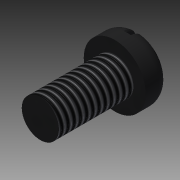
# Autodesk Inventor part: M3 6mm screw
Saved by Autodesk Inventor 2015 (Build 190159000, 159)
## iProperties
Created: 2015-10-31
Part Number: M3 6mm screw
Material: Nylon 6
Document SubType Name: Modeling
Designer: James
Density: 1.12 g/cm^3
Appearance: Nylon 6
Author: James
Autodesk Inventor part; units mm, degrees
ref_plane "YZ Plane" through (0, 0, 0) normal (1, 0, 0) x (0, 1, 0)
ref_plane "XZ Plane" through (0, 0, 0) normal (0, 1, 0) x (-1, 0, 0)
ref_plane "XY Plane" through (0, 0, 0) normal (0, 0, 1) x (1, 0, 0)
sketch "Sketch1" plane through (0, 0, 0) normal (0, 1, 0) x (-1, 0, 0)
  circle A0 centre (0, 0) radius 2.5
  dimension "d0" = 5
  constraints: 1 centre point, 1 coincident
  measures "d0" diameter of A0
extrude "Extrusion1" add sketch "Sketch1" along normal blind 2
fillet "Fillet1" radius 1 1 edges at (2.5, 2, 0)
sketch "Sketch2" plane through (0, 0, 0) normal (0, -1, 0) x (1, 0, 0)
  circle A0 centre (0, 0) radius 1.5
  constraints: 1 centre point, 1 coincident
extrude "Extrusion2" add sketch "Sketch2" along normal blind 6
thread "Thread1" size "M3x0.5" class "6g" standard "ANSI Metric M Profile" full length
sketch "Sketch3" plane through (0, 2, 0) normal (0, 1, 0) x (1, 0, 0)
  line L0 (-0.1996, -0.1996) -> (-0.1996, -1.4867)
  line L1 (-0.1996, 0.1996) -> (-0.1996, 1.4867)
  line L2 (0.1996, -0.1996) -> (0.1996, -1.4867)
  line L3 (0.1996, 0.1996) -> (0.1996, 1.4867)
  line L4 (-1.4867, -0.1996) -> (-0.1996, -0.1996)
  line L5 (0.1996, -0.1996) -> (1.4867, -0.1996)
  line L6 (-1.4867, 0.1996) -> (-0.1996, 0.1996)
  line L7 (0.1996, 0.1996) -> (1.4867, 0.1996)
  line L8 (0.1996, -1.4867) -> (0.1996, -2.6867)
  line L9 (0.1996, -2.6867) -> (-0.1996, -2.6867)
  line L10 (-0.1996, -2.6867) -> (-0.1996, -1.4867)
  line L11 (0.1996, 1.4867) -> (0.1996, 2.6867)
  line L12 (0.1996, 2.6867) -> (-0.1996, 2.6867)
  line L13 (-0.1996, 2.6867) -> (-0.1996, 1.4867)
  line L14 (1.4867, -0.1996) -> (1.4867, 0.1996)
  line L15 (-1.4867, -0.1996) -> (-1.4867, 0.1996)
  dimension "d15" = 1.2
  dimension "d16" = 1.2
  constraints: 32 end point, 5 vertical, 4 perpendicular, 1 collinear, 1 horizontal
  measures "d15" distance of L2.end L8.end
  measures "d16" distance of L3.end L11.end
extrude "Extrusion3" cut sketch "Sketch3" against normal blind 1
chamfer "Chamfer1" distance 0.1 angle 45 12 edges at (0.1996, 2, 0.8431) (0.1996, 1.7079, 2.1972) (-0.1996, 2, 0.8431) (-0.1996, 1.7079, 2.1972) (-0.8431, 2, 0.1996) (-0.8431, 2, -0.1996) (0.8431, 2, 0.1996) (0.8431, 2, -0.1996) (0.1996, 2, -0.8431) (0.1996, 1.7079, -2.1972) (-0.1996, 2, -0.8431) (-0.1996, 1.7079, -2.1972)
body "Solid1"
